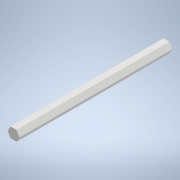
# Autodesk Inventor part: eje2_n
Saved by Autodesk Inventor 2022 (Build 260153000, 153)
## iProperties
Created: 2022-03-11
Part Number: eje2_n
Material: Generic
Document SubType Name: Modeling
Designer: katha
Density: 1 g/cm^3
Appearance: Default
Author: katha
Autodesk Inventor part; units mm, degrees
ref_plane "YZ Plane" through (0, 0, 0) normal (1, 0, 0) x (0, 1, 0)
ref_plane "XZ Plane" through (0, 0, 0) normal (0, 1, 0) x (-1, 0, 0)
ref_plane "XY Plane" through (0, 0, 0) normal (0, 0, 1) x (1, 0, 0)
sketch "Sketch1" plane through (0, 0, 0) normal (0, 0, 1) x (1, 0, 0)
  line L0 (0, 0) -> (3.1, 0) construction
  circle A0 centre (0, 0) radius 7.5 projected
  line L1 (0, 0) -> (1.55, 2.6847) construction
  line L2 (0, 0) -> (-1.55, 2.6847) construction
  line L3 (0, 0) -> (-3.1, 0) construction
  line L4 (0, 0) -> (-1.55, -2.6847) construction
  line L5 (0, 0) -> (1.55, -2.6847) construction
  line L6 (-1.55, 2.6847) -> (1.55, 2.6847)
  line L7 (1.55, 2.6847) -> (3.1, 0)
  line L8 (3.1, 0) -> (1.55, -2.6847)
  line L9 (1.55, -2.6847) -> (-1.55, -2.6847)
  line L10 (-1.55, -2.6847) -> (-3.1, 0)
  line L11 (-3.1, 0) -> (-1.55, 2.6847)
  line L12 (-1.7809, 3.0847) -> (1.7809, 3.0847) projected
  dimension "d0" = 3.1
  dimension "d3" = 360
  constraints: 24 end point, 2 horizontal, 2 parallel, 19 other
  measures "d0" distance of L0.start L0.end
extrude "Extrusion1" add sketch "Sketch1" against normal blind 80 contours L6 L7 L8 L9 L10 L11
sketch "Sketch2" plane through (-1.55, -2.6847, 0) normal (0, -1, 0) x (1, 0, 0)
  line L0 (0, 0) -> (0, -80) projected
  line L1 (3.1, 0) -> (3.1, -80) projected
  line L2 (106.9037, -80.1) -> (-63.0931, -80.1) projected
  ellipse E0 centre (1.709, -56.1) end of major axis (1.709, -55.45) minor radius 0.65 projected
  line L3 (1.709, -56.1) -> (-0.1699, -56.1) construction
  circle A0 centre (1.55, -56.1) radius 0.65
  line L4 (0, 0) -> (3.1, 0) projected
  circle A1 centre (1.55, -59.1) radius 0.65
  point P0 (1.55, 0)
  point P1 (1.55, 0)
  point P2 (1.6295, -55.4549)
  point P3 (1.6295, -56.7451)
  dimension "d7" = 1.3
  dimension "d8" = 56.1
  dimension "d9" = 3
  constraints: 2 centre point, 2 end point, 2 vertical alignment, 1 equal radius, 1 horizontal, 1 midpoint, 1 other
  measures "d7" diameter of A0
  measures "d8" distance from line of A0.centre L4
  measures "d9" distance of A1.centre A0.centre
extrude "Extrusion2" cut sketch "Sketch2" against normal blind 10 contours E0 A0 | A1 picked at (1.8134, -56.0482)
body "Solid1"
